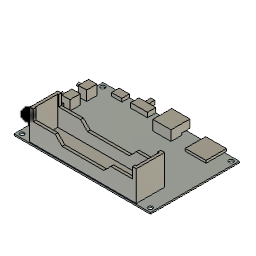
XAH-105 (Autodesk Fusion 360 design; units mm, degrees)
part number: 2025-10-06-10-12-29-326
Autodesk Fusion 360 part; units mm, degrees
sketch "Sketch1" plane through (0, 0, 0) normal (0, 0, 1) x (1, 0, 0)
sketch "Sketch2" plane through (0, 0, 0) normal (0, 0, 1) x (1, 0, 0)
  line L0 (49.015, -31.96) -> (-49.015, -31.96)
  line L1 (-49.015, -31.96) -> (-49.015, 31.96)
  line L2 (-49.015, 31.96) -> (49.015, 31.96)
  line L3 (49.015, 31.96) -> (49.015, -31.96)
  line L4 (49.015, -31.96) -> (-49.015, 31.96) construction
  line L5 (-49.015, -31.96) -> (49.015, 31.96) construction
  dimension "d1" = 98.03
  dimension "d2" = 63.92
  constraint horizontal L0
  constraint perpendicular L0 L1
  constraint parallel L0 L2
  constraint parallel L1 L3
  constraint coincident L4 origin
  constraint coincident L5 origin
  measures "d1" distance of L1.end L2.end
  measures "d2" distance of L0.end L1.end
extrude "Extrude1" add sketch "Sketch2" along normal blind 1.14
sketch "Sketch3" plane through (0, 0, 1.14) normal (0, 0, 1) x (-1, 0, 0)
  line L0 (-49.015, -31.96) -> (49.015, -31.96)
  line L1 (49.015, -31.96) -> (49.015, 31.96)
  line L2 (49.015, 31.96) -> (-49.015, 31.96)
  line L3 (-49.015, 31.96) -> (-49.015, -31.96)
  line L4 (-49.015, 31.96) -> (-38.345, 31.96) construction
  line L5 (49.015, 31.96) -> (38.345, 31.96) construction
  line L6 (38.345, 31.38) -> (38.345, 11.1)
  line L7 (38.345, 11.1) -> (-38.345, 11.1)
  line L8 (-38.345, 11.1) -> (-38.345, 31.38)
  line L9 (38.345, 31.96) -> (-38.345, 31.96)
  circle A0 centre (46.105, -28.98) radius 1.58
  circle A1 centre (46.105, 28.98) radius 1.58
  circle A2 centre (-46.035, -28.98) radius 1.58
  circle A3 centre (-46.035, 28.98) radius 1.58
  line L10 (38.345, 31.38) -> (-38.345, 31.38)
  dimension "d5" = 10.67
  dimension "d6" = 10.67
  dimension "d7" = 2.91
  dimension "d8" = 2.98
  dimension "d9" = 3.16
  dimension "d12" = 3.16
  dimension "d13" = 3.16
  dimension "d14" = 3.16
  dimension "d15" = 2.98
  dimension "d16" = 2.98
  dimension "d17" = 2.98
  dimension "d18" = 2.98
  dimension "d19" = 2.91
  dimension "d20" = 2.98
  dimension "d38" = 20.86
  dimension "d39" = 0.58
  constraint coincident L2.end L3.start
  constraint perpendicular L3 L4
  constraint coincident L1.end L2.start
  constraint perpendicular L1 L5
  constraint perpendicular L5 L6
  constraint perpendicular L6 L7
  constraint perpendicular L4 L8
  constraint perpendicular L8 L10
  measures "d5" distance of L2.end L4.end
  measures "d6" distance of L1.end L5.end
  measures "d7" distance of L1 A0.centre
  measures "d8" distance of L0 A0.centre
  measures "d9" diameter of A0
  measures "d12" diameter of A1
  measures "d13" diameter of A2
  measures "d14" diameter of A3
  measures "d15" distance of L3 A3.centre
  measures "d16" distance of L4 A3.centre
  measures "d17" distance of L3 A2.centre
  measures "d18" distance of L0 A2.centre
  measures "d19" distance of L1 A1.centre
  measures "d20" distance of L5 A1.centre
  measures "d38" distance of L5.end L6.end
  measures "d39" distance of L5.end L6.start
extrude "Extrude2" add sketch "Sketch3" along normal blind 21.58 contours L6 L7 L8 L10 | A0 | A1 | A2 | A3
sketch "Sketch5" plane through (0, 0, 1.14) normal (0, 0, 1) x (-1, 0, 0)
  circle A0 centre (46.105, 28.98) radius 1.58
  circle A1 centre (-46.035, -28.98) radius 1.58
  circle A2 centre (46.105, -28.98) radius 1.58
  circle A3 centre (-46.035, 28.98) radius 1.58
  line L0 (-49.015, -31.96) -> (49.015, -31.96)
  line L1 (49.015, -31.96) -> (49.015, 31.96)
  line L2 (49.015, 31.96) -> (-49.015, 31.96)
  line L3 (-49.015, 31.96) -> (-49.015, -31.96)
  line L4 (49.015, 31.96) -> (49.015, 21.71) construction
  line L5 (49.015, 21.71) -> (42.975, 21.71)
  line L6 (42.975, 21.71) -> (42.975, 14.26)
  line L7 (42.975, 14.26) -> (49.015, 14.26)
  line L8 (43.7525, 14.26) -> (43.7525, 9.51) construction
  line L9 (49.015, 9.74) -> (42.975, 9.74)
  line L10 (42.975, 9.74) -> (42.975, 2.29)
  line L11 (42.975, 2.29) -> (49.015, 2.29)
  line L12 (49.015, 2.29) -> (49.015, 9.74)
  line L13 (49.015, 9.74) -> (42.975, 9.74)
  line L14 (43.8683, 2.29) -> (43.8683, -2.46) construction
  line L15 (49.015, -2.23) -> (42.975, -2.23)
  line L16 (42.975, -2.23) -> (42.975, -9.68)
  line L17 (42.975, -9.68) -> (49.015, -9.68)
  line L18 (43.9024, -9.68) -> (43.9024, -14.43) construction
  line L19 (49.015, -14.2) -> (42.975, -14.2)
  line L20 (42.975, -14.2) -> (42.975, -21.65)
  line L21 (42.975, -21.65) -> (49.015, -21.65)
  line L22 (38.345, 11.1) -> (-38.345, 11.1)
  line L23 (-38.345, 11.1) -> (-38.345, 31.38)
  line L24 (-38.345, 31.38) -> (38.345, 31.38)
  line L25 (38.345, 31.38) -> (38.345, 11.1)
  dimension "d21" = 10.25
  dimension "d22" = 6.04
  dimension "d23" = 7.45
  dimension "d24" = 4.75
  dimension "d25" = 7.45
  dimension "d26" = 4.75
  dimension "d27" = 6.04
  dimension "d28" = 7.45
  dimension "d29" = 4.75
  dimension "d30" = 6.04
  dimension "d31" = 7.45
  dimension "d32" = 6.04
  dimension "d33" = 4.52
  dimension "d34" = 4.52
  dimension "d35" = 4.52
  constraint coincident L1.end L2.start
  constraint perpendicular L2 L4
  constraint perpendicular L4 L5
  constraint perpendicular L5 L6
  constraint coincident L1 L7.end
  constraint perpendicular L1 L7
  constraint coincident L7 L8.start
  constraint perpendicular L7 L8
  constraint coincident L1 L9.start
  constraint perpendicular L6 L9
  constraint perpendicular L9 L10
  constraint coincident L1 L11.end
  constraint perpendicular L1 L11
  constraint coincident L11 L14.start
  constraint perpendicular L11 L14
  constraint coincident L1 L15.start
  constraint perpendicular L14 L15
  constraint perpendicular L15 L16
  constraint coincident L1 L17.end
  constraint perpendicular L1 L17
  constraint coincident L17 L18.start
  constraint perpendicular L17 L18
  constraint coincident L1 L19.start
  constraint perpendicular L18 L19
  constraint perpendicular L19 L20
  constraint coincident L1 L21.end
  constraint perpendicular L1 L21
  measures "d21" distance of L1.end L4.end
  measures "d22" distance of L4.end L5.end
  measures "d23" distance of L5.end L6.end
  measures "d24" distance of L8.start L8.end
  measures "d25" distance of L9.end L10.end
  measures "d26" distance of L14.start L14.end
  measures "d27" distance of L15.start L15.end
  measures "d28" distance of L15.end L16.end
  measures "d29" distance of L18.start L18.end
  measures "d30" distance of L19.start L19.end
  measures "d31" distance of L19.end L20.end
  measures "d32" distance of L10 L12
  measures "d33" distance of L7 L9
  measures "d34" distance of L11 L15
  measures "d35" distance of L17 L19
extrude "Extrude3" add sketch "Sketch5" along normal blind 7.09 contours L1 L19 L20 L21 | L1 L5 L6 L7 | L1 L15 L16 L17 | L1 L9 L10 L11 L12 L13
extrude "Extrude4" cut 4 faces at (-45.3311, -29.4935, 22.72) (45.7717, -28.3669, 22.72) (45.7717, 29.5931, 22.72) (-45.3311, 28.4665, 22.72) along direction (0, 0, -1) blind 35
sketch "Sketch6" plane through (0, 0, 8.23) normal (0, 0, 1) x (-1, 0, 0)
  line L0 (42.975, 14.26) -> (49.015, 14.26)
  line L1 (49.015, 14.26) -> (49.015, 21.71)
  line L2 (49.015, 21.71) -> (42.975, 21.71)
  line L3 (42.975, 21.71) -> (42.975, 14.26)
  line L4 (49.015, 21.71) -> (46.905, 21.71) construction
  dimension "d42" = 2.11
  constraint coincident L1.end L2.start
  constraint perpendicular L1 L4
  measures "d42" distance of L1.end L4.end
shell "Shell1" thickness 2 removed faces 1 at (-12.7817, -17.86, 22.72)
sketch "Sketch7" plane through (0, -11.1, 0) normal (0, 1, 0) x (-1, 0, 0)
  line L0 (-38.345, 1.14) -> (38.345, 1.14)
  line L1 (38.345, 1.14) -> (38.345, 22.72)
  line L2 (38.345, 22.72) -> (-38.345, 22.72)
  line L3 (-38.345, 22.72) -> (-38.345, 1.14)
  line L4 (-35.5042, 22.72) -> (-35.5042, 15)
  line L5 (-35.5042, 15) -> (-20, 15)
  line L6 (-20, 15) -> (-15, 10)
  line L7 (-15, 10) -> (15, 10)
  line L8 (15, 10) -> (20, 15)
  line L9 (20, 15) -> (25, 15)
  line L10 (25, 15) -> (35.7465, 15)
  line L11 (35.7465, 15) -> (35.7465, 22.72)
  constraint coincident L2 L4.start
  constraint perpendicular L2 L4
  constraint perpendicular L4 L5
  constraint perpendicular L4 L7
  constraint perpendicular L6 L8
  constraint parallel L7 L9
  constraint parallel L9 L10
  constraint coincident L2 L11.end
  constraint perpendicular L2 L11
extrude "Extrude5" cut sketch "Sketch7" against normal blind 30 contours L2 L4 L5 L6 L7 L8 L9 L10 L11
sketch "Sketch8" plane through (0, -11.1, 0) normal (0, 1, 0) x (-1, 0, 0)
sketch "Sketch9" plane through (0, 0, 1.14) normal (0, 0, 1) x (-1, 0, 0)
  line L0 (42.975, -14.2) -> (49.015, -14.2)
  line L1 (49.015, -14.2) -> (49.015, -9.68)
  line L2 (49.015, -9.68) -> (42.975, -9.68)
  line L3 (42.975, -9.68) -> (42.975, -2.23)
  line L4 (42.975, -2.23) -> (49.015, -2.23)
  line L5 (49.015, -2.23) -> (49.015, 2.29)
  line L6 (49.015, 2.29) -> (42.975, 2.29)
  line L7 (42.975, 2.29) -> (42.975, 9.74)
  line L8 (42.975, 9.74) -> (49.015, 9.74)
  line L9 (49.015, 9.74) -> (49.015, 14.26)
  line L10 (49.015, 14.26) -> (42.975, 14.26)
  line L11 (42.975, 14.26) -> (42.975, 21.71)
  line L12 (42.975, 21.71) -> (49.015, 21.71)
  line L13 (49.015, 21.71) -> (49.015, 31.96)
  line L14 (49.015, 31.96) -> (-49.015, 31.96)
  line L15 (-49.015, 31.96) -> (-49.015, -31.96)
  line L16 (-49.015, -31.96) -> (49.015, -31.96)
  line L17 (49.015, -31.96) -> (49.015, -21.65)
  line L18 (49.015, -21.65) -> (42.975, -21.65)
  line L19 (42.975, -21.65) -> (42.975, -14.2)
  circle A0 centre (-46.035, -28.98) radius 1.58
  circle A1 centre (46.105, 28.98) radius 1.58
  circle A2 centre (-46.035, 28.98) radius 1.58
  circle A3 centre (46.105, -28.98) radius 1.58
  line L20 (38.345, 11.1) -> (-38.345, 11.1)
  line L21 (-38.345, 11.1) -> (-38.345, 31.38)
  line L22 (-38.345, 31.38) -> (38.345, 31.38)
  line L23 (38.345, 31.38) -> (38.345, 11.1)
  line L24 (-49.015, -31.96) -> (-38.335, -31.96) construction
  line L25 (-38.335, -31.96) -> (-38.335, -18.62)
  line L26 (-38.335, -18.62) -> (-23.405, -18.62)
  line L27 (-23.405, -18.62) -> (-23.405, -33.4)
  line L28 (-23.405, -33.4) -> (-38.335, -33.4)
  line L29 (-38.335, -33.4) -> (-38.335, -31.96)
  dimension "d46" = 10.68
  dimension "d47" = 13.34
  dimension "d48" = 14.93
  dimension "d49" = 14.78
  constraint coincident L15.end L16.start
  constraint perpendicular L15 L24
  constraint perpendicular L24 L25
  constraint perpendicular L25 L26
  constraint perpendicular L16 L27
  constraint perpendicular L25 L28
  constraint perpendicular L24 L29
  measures "d46" distance of L15.end L24.end
  measures "d47" distance of L24.end L25.end
  measures "d48" distance of L25.end L26.end
  measures "d49" distance of L26.end L27.end
extrude "Extrude6" add sketch "Sketch9" along normal blind 1.8 contours L16 L27 L28 L29 | L16 L25 L26 L27
sketch "Sketch10" plane through (0, 0, 1.14) normal (0, 0, 1) x (-1, 0, 0)
  line L0 (-23.405, -18.62) -> (-23.405, -31.96)
  line L1 (-23.405, -31.96) -> (49.015, -31.96)
  line L2 (49.015, -31.96) -> (49.015, -21.65)
  line L3 (49.015, -21.65) -> (42.975, -21.65)
  line L4 (42.975, -21.65) -> (42.975, -14.2)
  line L5 (42.975, -14.2) -> (49.015, -14.2)
  line L6 (49.015, -14.2) -> (49.015, -9.68)
  line L7 (49.015, -9.68) -> (42.975, -9.68)
  line L8 (42.975, -9.68) -> (42.975, -2.23)
  line L9 (42.975, -2.23) -> (49.015, -2.23)
  line L10 (49.015, -2.23) -> (49.015, 2.29)
  line L11 (49.015, 2.29) -> (42.975, 2.29)
  line L12 (42.975, 2.29) -> (42.975, 9.74)
  line L13 (42.975, 9.74) -> (49.015, 9.74)
  line L14 (49.015, 9.74) -> (49.015, 14.26)
  line L15 (49.015, 14.26) -> (42.975, 14.26)
  line L16 (42.975, 14.26) -> (42.975, 21.71)
  line L17 (42.975, 21.71) -> (49.015, 21.71)
  line L18 (49.015, 21.71) -> (49.015, 31.96)
  line L19 (49.015, 31.96) -> (-49.015, 31.96)
  line L20 (-49.015, 31.96) -> (-49.015, -31.96)
  line L21 (-49.015, -31.96) -> (-38.335, -31.96)
  line L22 (-38.335, -31.96) -> (-38.335, -18.62)
  line L23 (-38.335, -18.62) -> (-23.405, -18.62)
  circle A0 centre (-46.035, -28.98) radius 1.58
  circle A1 centre (46.105, 28.98) radius 1.58
  circle A2 centre (-46.035, 28.98) radius 1.58
  circle A3 centre (46.105, -28.98) radius 1.58
  line L24 (38.345, 11.1) -> (-38.345, 11.1)
  line L25 (-38.345, 11.1) -> (-38.345, 31.38)
  line L26 (-38.345, 31.38) -> (38.345, 31.38)
  line L27 (38.345, 31.38) -> (38.345, 11.1)
  line L28 (-23.405, -27.6756) -> (-12.205, -27.6756) construction
  line L29 (-12.205, -31.96) -> (-12.205, -33.27)
  line L30 (-12.205, -33.27) -> (0.895, -33.27)
  line L31 (0.895, -33.27) -> (0.895, -19.63)
  line L32 (0.895, -19.63) -> (-12.205, -19.63)
  line L33 (-12.205, -19.63) -> (-12.205, -33.27)
  dimension "d52" = 11.2
  dimension "d53" = 1.31
  dimension "d54" = 13.1
  dimension "d55" = 13.64
  constraint coincident L0 L28.start
  constraint perpendicular L0 L28
  constraint coincident L1 L29.start
  constraint perpendicular L1 L29
  constraint perpendicular L29 L30
  constraint perpendicular L1 L31
  constraint perpendicular L29 L32
  constraint perpendicular L30 L33
  measures "d52" distance of L28.start L28.end
  measures "d53" distance of L29.start L29.end
  measures "d54" distance of L29.end L30.end
  measures "d55" distance of L30.end L31.end
extrude "Extrude7" add sketch "Sketch10" along normal blind 7.22 contours L1 L31 L32 L33 | L1 L29 L30 L31 L33
sketch "Sketch11" plane through (0, 33.27, 0) normal (0, 1, 0) x (-1, 0, 0)
  line L0 (-12.205, 1.14) -> (0.895, 1.14)
  line L1 (0.895, 1.14) -> (0.895, 8.36)
  line L2 (0.895, 8.36) -> (-12.205, 8.36)
  line L3 (-12.205, 8.36) -> (-12.205, 1.14)
  line L4 (0.895, 1.14) -> (0.895, 2.49) construction
  line L5 (0.895, 2.49) -> (-12.205, 2.49)
  dimension "d58" = 1.35
  constraint coincident L0.end L1.start
  constraint perpendicular L0 L4
  constraint coincident L3 L5.end
  constraint perpendicular L3 L5
  measures "d58" distance of L0.end L4.end
extrude "Extrude8" cut sketch "Sketch11" against normal blind 6 contours L0 L1 L3 L5
sketch "Sketch12" plane through (0, 0, 1.14) normal (0, 0, 1) x (-1, 0, 0)
  line L0 (-12.205, -27.27) -> (-12.205, -19.63)
  line L1 (-12.205, -19.63) -> (0.895, -19.63)
  line L2 (0.895, -19.63) -> (0.895, -27.27)
  line L3 (0.895, -27.27) -> (-12.205, -27.27)
  line L4 (-23.405, -31.96) -> (49.015, -31.96)
  line L5 (49.015, -31.96) -> (49.015, -21.65)
  line L6 (49.015, -21.65) -> (42.975, -21.65)
  line L7 (42.975, -21.65) -> (42.975, -14.2)
  line L8 (42.975, -14.2) -> (49.015, -14.2)
  line L9 (49.015, -14.2) -> (49.015, -9.68)
  line L10 (49.015, -9.68) -> (42.975, -9.68)
  line L11 (42.975, -9.68) -> (42.975, -2.23)
  line L12 (42.975, -2.23) -> (49.015, -2.23)
  line L13 (49.015, -2.23) -> (49.015, 2.29)
  line L14 (49.015, 2.29) -> (42.975, 2.29)
  line L15 (42.975, 2.29) -> (42.975, 9.74)
  line L16 (42.975, 9.74) -> (49.015, 9.74)
  line L17 (49.015, 9.74) -> (49.015, 14.26)
  line L18 (49.015, 14.26) -> (42.975, 14.26)
  line L19 (42.975, 14.26) -> (42.975, 21.71)
  line L20 (42.975, 21.71) -> (49.015, 21.71)
  line L21 (49.015, 21.71) -> (49.015, 31.96)
  line L22 (49.015, 31.96) -> (-49.015, 31.96)
  line L23 (-49.015, 31.96) -> (-49.015, -31.96)
  line L24 (-49.015, -31.96) -> (-38.335, -31.96)
  line L25 (-38.335, -31.96) -> (-38.335, -18.62)
  line L26 (-38.335, -18.62) -> (-23.405, -18.62)
  line L27 (-23.405, -18.62) -> (-23.405, -31.96)
  circle A0 centre (-46.035, -28.98) radius 1.58
  circle A1 centre (46.105, 28.98) radius 1.58
  circle A2 centre (-46.035, 28.98) radius 1.58
  circle A3 centre (46.105, -28.98) radius 1.58
  line L28 (38.345, 11.1) -> (-38.345, 11.1)
  line L29 (-38.345, 11.1) -> (-38.345, 31.38)
  line L30 (-38.345, 31.38) -> (38.345, 31.38)
  line L31 (38.345, 31.38) -> (38.345, 11.1)
  line L32 (0.895, -27.27) -> (10.995, -27.27) construction
  line L33 (10.995, -31.96) -> (10.995, -25.92)
  line L34 (10.995, -25.92) -> (23.085, -25.92)
  line L35 (23.085, -25.92) -> (23.085, -31.96)
  line L36 (23.085, -31.96) -> (10.995, -31.96)
  dimension "d61" = 10.1
  dimension "d62" = 6.04
  dimension "d63" = 12.09
  constraint coincident L2.end L3.start
  constraint perpendicular L2 L32
  constraint coincident L4 L33.start
  constraint perpendicular L4 L33
  constraint perpendicular L33 L34
  constraint coincident L4 L35.end
  constraint perpendicular L4 L35
  measures "d61" distance of L2.end L32.end
  measures "d62" distance of L33.start L33.end
  measures "d63" distance of L33.end L34.end
extrude "Extrude9" add sketch "Sketch12" along normal blind 3.4 contours L4 L33 L34 L35 L36
extrude "Extrude10" add 1 faces at (-15.025, 27.9333, 4.54) along direction (0, 0, -1) blind 5.43
sketch "Sketch13" plane through (0, 31.96, 0) normal (0, 1, 0) x (-1, 0, 0)
  line L0 (10.995, 1.14) -> (-23.405, 1.14)
  line L1 (-23.405, 1.14) -> (-38.335, 1.14)
  line L2 (-38.335, 1.14) -> (-49.015, 1.14)
  line L3 (-49.015, 1.14) -> (-49.015, 0)
  line L4 (-49.015, 0) -> (10.995, 0)
  line L5 (10.995, 0) -> (10.995, -0.89)
  line L6 (10.995, -0.89) -> (23.085, -0.89)
  line L7 (23.085, -0.89) -> (23.085, 0)
  line L8 (23.085, 0) -> (49.015, 0)
  line L9 (49.015, 0) -> (49.015, 1.14)
  line L10 (49.015, 1.14) -> (23.085, 1.14)
  line L11 (23.085, 1.14) -> (23.085, 4.54)
  line L12 (23.085, 4.54) -> (10.995, 4.54)
  line L13 (10.995, 4.54) -> (10.995, 1.14)
  line L14 (17.265, 3.09) -> (20.195, 3.09)
  line L15 (20.195, 3.09) -> (20.195, 0.15)
  line L16 (20.195, 0.15) -> (17.265, 0.15)
  line L17 (17.265, 0.15) -> (17.265, 3.09)
  dimension "d68" = 2.93
  dimension "d69" = 2.94
  dimension "d70" = 1.45
  dimension "d71" = 2.89
  constraint horizontal L14
  constraint vertical L15
  constraint horizontal L16
  constraint vertical L17
  measures "d68" distance of L14.start L14.end
  measures "d69" distance of L14.start L16.end
  measures "d70" distance of L12 L14
  measures "d71" distance of L11 L15
extrude "Extrude11" add sketch "Sketch13" along normal blind 5.6 contours L14 L15 L16 L17
sketch "Sketch14" plane through (0, 0, 1.14) normal (0, 0, 1) x (-1, 0, 0)
  line L0 (38.345, 11.1) -> (-38.345, 11.1)
  line L1 (-38.345, 11.1) -> (-38.345, 31.38)
  line L2 (-38.345, 31.38) -> (38.345, 31.38)
  line L3 (38.345, 31.38) -> (38.345, 11.1)
  circle A0 centre (46.105, -28.98) radius 1.58
  circle A1 centre (-46.035, 28.98) radius 1.58
  circle A2 centre (46.105, 28.98) radius 1.58
  circle A3 centre (-46.035, -28.98) radius 1.58
  line L4 (10.995, -31.96) -> (10.995, -25.92)
  line L5 (10.995, -25.92) -> (23.085, -25.92)
  line L6 (23.085, -25.92) -> (23.085, -31.96)
  line L7 (23.085, -31.96) -> (49.015, -31.96)
  line L8 (49.015, -31.96) -> (49.015, -21.65)
  line L9 (49.015, -21.65) -> (42.975, -21.65)
  line L10 (42.975, -21.65) -> (42.975, -14.2)
  line L11 (42.975, -14.2) -> (49.015, -14.2)
  line L12 (49.015, -14.2) -> (49.015, -9.68)
  line L13 (49.015, -9.68) -> (42.975, -9.68)
  line L14 (42.975, -9.68) -> (42.975, -2.23)
  line L15 (42.975, -2.23) -> (49.015, -2.23)
  line L16 (49.015, -2.23) -> (49.015, 2.29)
  line L17 (49.015, 2.29) -> (42.975, 2.29)
  line L18 (42.975, 2.29) -> (42.975, 9.74)
  line L19 (42.975, 9.74) -> (49.015, 9.74)
  line L20 (49.015, 9.74) -> (49.015, 14.26)
  line L21 (49.015, 14.26) -> (42.975, 14.26)
  line L22 (42.975, 14.26) -> (42.975, 21.71)
  line L23 (42.975, 21.71) -> (49.015, 21.71)
  line L24 (49.015, 21.71) -> (49.015, 31.96)
  line L25 (49.015, 31.96) -> (-49.015, 31.96)
  line L26 (-49.015, 31.96) -> (-49.015, -31.96)
  line L27 (-49.015, -31.96) -> (-38.335, -31.96)
  line L28 (-38.335, -31.96) -> (-38.335, -18.62)
  line L29 (-38.335, -18.62) -> (-23.405, -18.62)
  line L30 (-23.405, -18.62) -> (-23.405, -31.96)
  line L31 (-23.405, -31.96) -> (10.995, -31.96)
  line L32 (-12.205, -27.27) -> (-12.205, -19.63)
  line L33 (-12.205, -19.63) -> (0.895, -19.63)
  line L34 (0.895, -19.63) -> (0.895, -27.27)
  line L35 (0.895, -27.27) -> (-12.205, -27.27)
  line L36 (23.085, -28.94) -> (29.935, -28.94) construction
  line L37 (29.935, -31.96) -> (37.335, -31.96)
  line L38 (37.335, -31.96) -> (37.335, -26.46)
  line L39 (29.935, -26.46) -> (37.335, -26.46)
  line L40 (29.935, -26.46) -> (29.935, -31.96)
  dimension "d74" = 6.85
  dimension "d75" = 7.4
  dimension "d76" = 5.5
  constraint midpoint L6 L36.start
  constraint perpendicular L6 L36
  constraint coincident L7 L37.start
  constraint parallel L7 L37
  constraint perpendicular L37 L38
  constraint perpendicular L38 L39
  constraint perpendicular L7 L40
  measures "d74" distance of L36.start L36.end
  measures "d75" distance of L37.start L37.end
  measures "d76" distance of L37.end L38.end
extrude "Extrude12" add sketch "Sketch14" along normal blind 2.3 contours L7 L37 L38 L39 L40
sketch "Sketch15" plane through (0, 0, 1.14) normal (0, 0, 1) x (-1, 0, 0)
  line L0 (37.335, -26.46) -> (37.335, -31.96)
  line L1 (37.335, -31.96) -> (49.015, -31.96)
  line L2 (49.015, -31.96) -> (49.015, -21.65)
  line L3 (49.015, -21.65) -> (42.975, -21.65)
  line L4 (42.975, -21.65) -> (42.975, -14.2)
  line L5 (42.975, -14.2) -> (49.015, -14.2)
  line L6 (49.015, -14.2) -> (49.015, -9.68)
  line L7 (49.015, -9.68) -> (42.975, -9.68)
  line L8 (42.975, -9.68) -> (42.975, -2.23)
  line L9 (42.975, -2.23) -> (49.015, -2.23)
  line L10 (49.015, -2.23) -> (49.015, 2.29)
  line L11 (49.015, 2.29) -> (42.975, 2.29)
  line L12 (42.975, 2.29) -> (42.975, 9.74)
  line L13 (42.975, 9.74) -> (49.015, 9.74)
  line L14 (49.015, 9.74) -> (49.015, 14.26)
  line L15 (49.015, 14.26) -> (42.975, 14.26)
  line L16 (42.975, 14.26) -> (42.975, 21.71)
  line L17 (42.975, 21.71) -> (49.015, 21.71)
  line L18 (49.015, 21.71) -> (49.015, 31.96)
  line L19 (49.015, 31.96) -> (-49.015, 31.96)
  line L20 (-49.015, 31.96) -> (-49.015, -31.96)
  line L21 (-49.015, -31.96) -> (-38.335, -31.96)
  line L22 (-38.335, -31.96) -> (-38.335, -18.62)
  line L23 (-38.335, -18.62) -> (-23.405, -18.62)
  line L24 (-23.405, -18.62) -> (-23.405, -31.96)
  line L25 (-23.405, -31.96) -> (10.995, -31.96)
  line L26 (10.995, -31.96) -> (10.995, -25.92)
  line L27 (10.995, -25.92) -> (23.085, -25.92)
  line L28 (23.085, -25.92) -> (23.085, -31.96)
  line L29 (23.085, -31.96) -> (29.935, -31.96)
  line L30 (29.935, -31.96) -> (29.935, -26.46)
  line L31 (29.935, -26.46) -> (37.335, -26.46)
  line L32 (38.345, 11.1) -> (-38.345, 11.1)
  line L33 (-38.345, 11.1) -> (-38.345, 31.38)
  line L34 (-38.345, 31.38) -> (38.345, 31.38)
  line L35 (38.345, 31.38) -> (38.345, 11.1)
  circle A0 centre (46.105, -28.98) radius 1.58
  circle A1 centre (-46.035, 28.98) radius 1.58
  circle A2 centre (46.105, 28.98) radius 1.58
  circle A3 centre (-46.035, -28.98) radius 1.58
  line L36 (-12.205, -27.27) -> (-12.205, -19.63)
  line L37 (-12.205, -19.63) -> (0.895, -19.63)
  line L38 (0.895, -19.63) -> (0.895, -27.27)
  line L39 (0.895, -27.27) -> (-12.205, -27.27)
sketch "Sketch16" plane through (0, 0, 1.14) normal (0, 0, 1) x (1, 0, 0)
sketch "Sketch17" plane through (-49.015, 0, 0) normal (-1, 0, 0) x (0, -1, 0)
  line L0 (-31.96, 0) -> (31.96, 0)
  line L1 (31.96, 0) -> (31.96, 1.14)
  line L2 (31.96, 1.14) -> (21.71, 1.14)
  line L3 (21.71, 1.14) -> (21.71, 8.23)
  line L4 (21.71, 8.23) -> (14.26, 8.23)
  line L5 (14.26, 8.23) -> (14.26, 1.14)
  line L6 (14.26, 1.14) -> (9.74, 1.14)
  line L7 (9.74, 1.14) -> (9.74, 8.23)
  line L8 (9.74, 8.23) -> (2.29, 8.23)
  line L9 (2.29, 8.23) -> (2.29, 1.14)
  line L10 (2.29, 1.14) -> (-2.23, 1.14)
  line L11 (-2.23, 1.14) -> (-2.23, 8.23)
  line L12 (-2.23, 8.23) -> (-9.68, 8.23)
  line L13 (-9.68, 8.23) -> (-9.68, 1.14)
  line L14 (-9.68, 1.14) -> (-14.2, 1.14)
  line L15 (-14.2, 1.14) -> (-14.2, 8.23)
  line L16 (-14.2, 8.23) -> (-21.65, 8.23)
  line L17 (-21.65, 8.23) -> (-21.65, 1.14)
  line L18 (-21.65, 1.14) -> (-31.96, 1.14)
  line L19 (-31.96, 1.14) -> (-31.96, 0)
  circle A0 centre (-6, 5.08) radius 1.69
  circle A1 centre (-18, 5.08) radius 1.69
  circle A2 centre (6, 5.08) radius 1.69
  circle A3 centre (18, 5.08) radius 1.69
  line L20 (14.26, 8.23) -> (21.71, 8.23)
  dimension "d79" = 3.38
  dimension "d80" = 3.38
  dimension "d81" = 3.38
  dimension "d82" = 3.38
  dimension "d83" = 3.15
  dimension "d84" = 3.15
  dimension "d85" = 3.15
  dimension "d86" = 3.15
  measures "d79" diameter of A0
  measures "d80" diameter of A1
  measures "d81" diameter of A2
  measures "d82" diameter of A3
  measures "d83" distance of L16 A1.centre
  measures "d84" distance of L12 A0.centre
  measures "d85" distance of L8 A2.centre
  measures "d86" distance of A3.centre L20
extrude "Extrude13" add sketch "Sketch17" along normal blind 3.7 draft -6 contours A0 | A1 | A2 | A3
